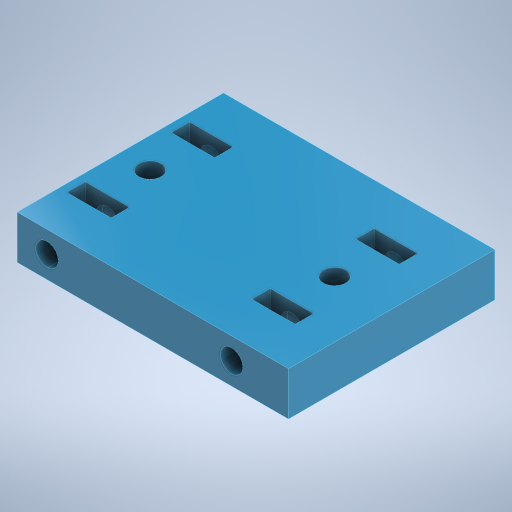
# Autodesk Inventor part: 3D_upper_to_head1
Saved by Autodesk Inventor 2024 (Build 280153000, 153)
## iProperties
Created: 2024-09-08
Part Number: 3D_upper_to_head1
Material: 일반
Document SubType Name: Modeling
Designer: jmha0
Density: 1 g/cm^3
Appearance: 하늘색 짙음
Author: jmha0
Autodesk Inventor part; units mm, degrees
ref_plane "YZ Plane" through (0, 0, 0) normal (1, 0, 0) x (0, 1, 0)
ref_plane "XZ Plane" through (0, 0, 0) normal (0, 1, 0) x (-1, 0, 0)
ref_plane "XY Plane" through (0, 0, 0) normal (0, 0, 1) x (1, 0, 0)
sketch "스케치1" plane through (0, 0, 0) normal (0, 1, 0) x (-1, 0, 0)
  line L0 (206.554, -381.1375) -> (206.9537, -381.1375)
  line L1 (206.9537, -381.1375) -> (207.1542, -381.1375)
  line L2 (207.1542, -381.1375) -> (210.304, -381.1375)
  line L3 (210.304, -381.1375) -> (210.304, -370.6375)
  line L4 (210.304, -370.6375) -> (211.404, -370.6375)
  line L5 (211.404, -370.6375) -> (211.404, -356.1375)
  line L6 (211.404, -356.1375) -> (224.204, -356.1375)
  line L7 (224.204, -370.6375) -> (224.204, -356.1375)
  line L8 (224.204, -370.6375) -> (225.304, -370.6375)
  line L9 (225.304, -381.1375) -> (225.304, -370.6375)
  line L10 (225.304, -381.1375) -> (228.9537, -381.1375)
  line L11 (228.9537, -381.1375) -> (229.1542, -381.1375)
  line L12 (229.1542, -381.1375) -> (233.029, -381.1375)
  line L13 (233.029, -383.6375) -> (233.029, -381.1375)
  line L14 (233.029, -383.6375) -> (247.079, -383.6375)
  line L15 (247.079, -383.6375) -> (247.079, -381.1375)
  line L16 (247.079, -381.1375) -> (250.9537, -381.1375)
  line L17 (250.9537, -381.1375) -> (251.1542, -381.1375)
  line L18 (251.1542, -381.1375) -> (255.029, -381.1375)
  line L19 (255.029, -383.6375) -> (255.029, -381.1375)
  line L20 (255.029, -383.6375) -> (258.054, -383.6375)
  line L21 (258.054, -353.6375) -> (258.054, -383.6375)
  line L22 (255.029, -353.6375) -> (258.054, -353.6375)
  line L23 (255.029, -353.6375) -> (255.029, -356.1375)
  line L24 (251.1542, -356.1375) -> (255.029, -356.1375)
  line L25 (250.9537, -356.1375) -> (251.1542, -356.1375)
  line L26 (247.079, -356.1375) -> (250.9537, -356.1375)
  line L27 (247.079, -353.6375) -> (247.079, -356.1375)
  line L28 (233.029, -353.6375) -> (247.079, -353.6375)
  line L29 (233.029, -353.6375) -> (233.029, -356.1375)
  line L30 (229.1542, -356.1375) -> (233.029, -356.1375)
  line L31 (228.9537, -356.1375) -> (229.1542, -356.1375)
  line L32 (225.079, -356.1375) -> (228.9537, -356.1375)
  line L33 (225.079, -353.6375) -> (225.079, -356.1375)
  line L34 (211.029, -353.6375) -> (225.079, -353.6375)
  line L35 (211.029, -353.6375) -> (211.029, -356.1375)
  line L36 (207.1542, -356.1375) -> (211.029, -356.1375)
  line L37 (206.9537, -356.1375) -> (207.1542, -356.1375)
  line L38 (206.554, -356.1375) -> (206.9537, -356.1375)
  line L39 (206.554, -356.1375) -> (206.554, -381.1375)
  circle A0 centre (240.054, -368.6375) radius 5.2901
  line L40 (258.054, -356.1375) -> (225.304, -356.1375)
  line L41 (225.304, -356.1375) -> (225.304, -381.1375)
  line L42 (225.304, -381.1375) -> (258.054, -381.1375)
  line L43 (258.054, -381.1375) -> (258.054, -356.1375)
  line L44 (257.854, -356.3375) -> (225.504, -356.3375)
  line L45 (225.504, -356.3375) -> (225.504, -380.9375)
  line L46 (225.504, -380.9375) -> (257.854, -380.9375)
  line L47 (257.854, -380.9375) -> (257.854, -356.3375)
  line L48 (255.029, -354.8875) -> (251.054, -354.8875)
  circle A1 centre (251.054, -354.8875) radius 0.8707
  line L49 (255.029, -382.3875) -> (247.079, -382.3875)
  line L50 (251.054, -354.8875) -> (251.054, -382.3875)
  line L51 (233.029, -354.8875) -> (229.054, -354.8875)
  line L52 (229.054, -354.8875) -> (229.054, -382.3875)
  dimension "d37" = 25
  dimension "d38" = 32.75
  dimension "d39" = 0.2
  dimension "d40" = 2.5
  dimension "d41" = 7.95
  dimension "d42" = 3.975
  dimension "d43" = 3.975
  constraints: 106 end point, 5 midpoint, 5 parallel, 3 perpendicular, 2 centre point, 2 horizontal, 1 coincident, 1 point on line, 3 other
  measures "d37" distance of L18.end L24.end
  measures "d38" distance from line of L21 L9.start
  measures "d39" distance between parallel lines of L43 L47
  measures "d40" distance of L22.start L24.end
  measures "d41" distance between parallel lines of L27 L23
  measures "d42" distance of L48.start L48.end
  measures "d43" distance of L51.start L51.end
extrude "돌출2" add sketch "스케치1" along normal blind 5.2 contours L52 L46 L45 L44 | L44 L50 L46 L52 | L44 L47 L46 L50 | A0
sketch "스케치4" plane through (-225.504, 0, -380.9375) normal (0, 0, -1) x (-1, 0, 0)
  line L0 (0, 0) -> (32.35, 0) projected
  line L1 (32.35, 0) -> (32.35, 5.2) projected
  line L2 (0, 5.2) -> (32.35, 5.2) projected
  line L3 (0, 0) -> (0, 5.2) projected
  line L4 (32.35, 5.2) -> (28.8, 5.2)
  line L5 (32.35, 5.2) -> (0, 5.2) projected
  line L6 (0, 5.2) -> (6.8, 5.2)
  line L7 (32.35, 2.6) -> (0, 2.6)
  circle A0 centre (28.8, 2.6) radius 1.35
  circle A1 centre (6.8, 2.6) radius 1.35
  point P0 (-225.504, 0)
  dimension "d59" = 3.55
  dimension "d60" = 6.8
  dimension "d69" = 2.7
  dimension "d70" = 2.7
  constraints: 6 end point, 4 point on line, 2 centre point, 2 midpoint
  measures "d59" distance of L1.end L4.end
  measures "d60" distance of L2.start L6.end
  measures "d69" diameter of A0
  measures "d70" diameter of A1
extrude "돌출3" cut sketch "스케치4" against normal blind 8 contours A1 L7 | L7 A1 | A0 L7 | L7 A0
sketch "스케치5" plane through (-257.854, 0, -356.3375) normal (0, 0, 1) x (1, 0, 0)
  circle A0 centre (3.55, 3) radius 1.35 projected
  circle A1 centre (25.55, 3) radius 1.35 projected
  circle A2 centre (3.55, 2.6) radius 1.35 projected
  circle A3 centre (25.55, 2.6) radius 1.35 projected
  point P0 (257.854, 0)
extrude "돌출4" cut sketch "스케치5" against normal blind 8 contours A2 A0 | A0 A2 | A3 A1 | A1 A3 picked at (3.4443, 2.4292) picked at (3.7277, 1.535) picked at (25.4443, 2.4292) picked at (25.7277, 1.535)
sketch "스케치6" plane through (0, 0, 0) normal (0, -1, 0) x (1, 0, 0)
  line L0 (-225.504, -356.3375) -> (-225.504, -380.9375) projected
  line L1 (-225.504, -356.3375) -> (-225.504, -380.9375) projected
  line L2 (-225.504, -356.3375) -> (-225.504, -380.9375) projected
  line L3 (-225.504, -356.3375) -> (-225.504, -380.9375) projected
  line L4 (-257.854, -356.3375) -> (-225.504, -356.3375) projected
  line L5 (-230.954, -380.9375) -> (-233.654, -380.9375) projected
  line L6 (-230.954, -372.9375) -> (-233.654, -372.9375) projected
  line L7 (-233.654, -356.3375) -> (-230.954, -356.3375) projected
  line L8 (-233.654, -364.3375) -> (-230.954, -364.3375) projected
  line L9 (-230.954, -372.9375) -> (-233.654, -372.9375) projected
  line L10 (-230.954, -372.9375) -> (-233.654, -372.9375) projected
  line L11 (-230.954, -380.9375) -> (-233.654, -380.9375) projected
  line L12 (-233.654, -364.3375) -> (-230.954, -364.3375) projected
  line L13 (-233.654, -364.3375) -> (-230.954, -364.3375) projected
  line L14 (-233.654, -356.3375) -> (-230.954, -356.3375) projected
  line L15 (-255.654, -356.3375) -> (-252.954, -356.3375) projected
  line L16 (-255.654, -364.3375) -> (-252.954, -364.3375) projected
  line L17 (-255.654, -356.3375) -> (-252.954, -356.3375) projected
  line L18 (-257.854, -356.3375) -> (-225.504, -356.3375) projected
  line L19 (-257.854, -380.9375) -> (-257.854, -356.3375) projected
  line L20 (-257.854, -380.9375) -> (-257.854, -356.3375) projected
  line L21 (-257.854, -356.3375) -> (-225.504, -356.3375) projected
  line L22 (-257.854, -380.9375) -> (-257.854, -356.3375) projected
  line L23 (-225.504, -380.9375) -> (-257.854, -380.9375) projected
  line L24 (-225.504, -356.3375) -> (-225.504, -380.9375) projected
  line L25 (-257.854, -356.3375) -> (-225.504, -356.3375) projected
  line L26 (-225.504, -356.3375) -> (-225.504, -380.9375) projected
  line L27 (-225.504, -380.9375) -> (-257.854, -380.9375) projected
  line L28 (-257.854, -380.9375) -> (-257.854, -356.3375) projected
  line L29 (-257.854, -356.3375) -> (-225.504, -356.3375) projected
  line L30 (-257.854, -356.3375) -> (-225.504, -356.3375) projected
  line L31 (-257.854, -380.9375) -> (-257.854, -356.3375) projected
  line L32 (-257.854, -380.9375) -> (-257.854, -356.3375) projected
  line L33 (-255.654, -364.3375) -> (-252.954, -364.3375) projected
  line L34 (-255.654, -364.3375) -> (-252.954, -364.3375) projected
  line L35 (-252.954, -372.9375) -> (-255.654, -372.9375) projected
  line L36 (-252.954, -372.9375) -> (-255.654, -372.9375) projected
  line L37 (-252.954, -372.9375) -> (-255.654, -372.9375) projected
  line L38 (-252.954, -380.9375) -> (-255.654, -380.9375) projected
  line L39 (-252.954, -380.9375) -> (-255.654, -380.9375) projected
  line L40 (-225.504, -380.9375) -> (-257.854, -380.9375) projected
  line L41 (-225.504, -380.9375) -> (-257.854, -380.9375) projected
  line L42 (-225.504, -380.9375) -> (-257.854, -380.9375) projected
  line L43 (-225.504, -380.9375) -> (-257.854, -380.9375) projected
  line L44 (-252.954, -356.3375) -> (-252.954, -364.3375) projected
  line L45 (-255.654, -356.3375) -> (-255.654, -364.3375) projected
  line L46 (-255.654, -380.9375) -> (-255.654, -372.9375) projected
  line L47 (-252.954, -380.9375) -> (-252.954, -372.9375) projected
  line L48 (-233.654, -380.9375) -> (-233.654, -372.9375) projected
  line L49 (-230.954, -380.9375) -> (-230.954, -372.9375) projected
  line L50 (-233.654, -356.3375) -> (-233.654, -364.3375) projected
  line L51 (-230.954, -356.3375) -> (-230.954, -364.3375) projected
  line L52 (-232.304, -365.7508) -> (-231.054, -366.4725)
  line L53 (-233.554, -366.4725) -> (-232.304, -365.7508)
  line L54 (-229.804, -367.1941) -> (-229.804, -368.6375)
  line L55 (-231.054, -366.4725) -> (-229.804, -367.1941)
  line L56 (-234.804, -368.6375) -> (-234.804, -367.1941)
  line L57 (-234.804, -367.1941) -> (-233.554, -366.4725)
  line L58 (-234.804, -368.6375) -> (-234.804, -367.1941)
  line L59 (-234.804, -370.0809) -> (-234.804, -368.6375)
  line L60 (-231.054, -370.8026) -> (-232.304, -371.5243)
  line L61 (-232.304, -371.5243) -> (-233.554, -370.8026)
  line L62 (-229.804, -368.6375) -> (-229.804, -370.0809)
  line L63 (-229.804, -370.0809) -> (-231.054, -370.8026)
  line L64 (-229.804, -367.1941) -> (-229.804, -368.6375)
  line L65 (-231.054, -366.4725) -> (-229.804, -367.1941)
  line L66 (-233.554, -370.8026) -> (-234.804, -370.0809)
  line L67 (-234.804, -370.0809) -> (-234.804, -368.6375)
  line L68 (-254.304, -365.7508) -> (-253.054, -366.4725)
  line L69 (-255.554, -366.4725) -> (-254.304, -365.7508)
  line L70 (-251.804, -367.1941) -> (-251.804, -368.6375)
  line L71 (-253.054, -366.4725) -> (-251.804, -367.1941)
  line L72 (-256.804, -368.6375) -> (-256.804, -367.1941)
  line L73 (-256.804, -367.1941) -> (-255.554, -366.4725)
  line L74 (-256.804, -368.6375) -> (-256.804, -367.1941)
  line L75 (-256.804, -370.0809) -> (-256.804, -368.6375)
  line L76 (-253.054, -370.8026) -> (-254.304, -371.5243)
  line L77 (-254.304, -371.5243) -> (-255.554, -370.8026)
  line L78 (-251.804, -368.6375) -> (-251.804, -370.0809)
  line L79 (-251.804, -370.0809) -> (-253.054, -370.8026)
  line L80 (-251.804, -367.1941) -> (-251.804, -368.6375)
  line L81 (-253.054, -366.4725) -> (-251.804, -367.1941)
  line L82 (-255.554, -370.8026) -> (-256.804, -370.0809)
  line L83 (-256.804, -370.0809) -> (-256.804, -368.6375)
  point P0 (0, 0)
  point P1 (-232.304, -368.6375)
  point P2 (-254.304, -368.6375)
  dimension "d75" = 5.7735
  constraints: 64 end point, 4 other
  measures "d75" distance of L68.start L77.start
extrude "돌출5" cut sketch "스케치6" against normal blind 2 contours L52 L55 L54 L62 L63 L60 L61 L66 L59 L56 L57 L53 | L68 L71 L70 L78 L79 L76 L77 L82 L75 L72 L73 L69
sketch "스케치7" plane through (0, 2, 0) normal (0, -1, 0) x (1, 0, 0)
  line L0 (-256.804, -367.1941) -> (-254.304, -365.7508) projected
  line L1 (-256.804, -370.0809) -> (-256.804, -367.1941) projected
  line L2 (-254.304, -371.5243) -> (-256.804, -370.0809) projected
  line L3 (-251.804, -370.0809) -> (-254.304, -371.5243) projected
  line L4 (-251.804, -367.1941) -> (-251.804, -370.0809) projected
  line L5 (-254.304, -365.7508) -> (-251.804, -367.1941) projected
  line L6 (-234.804, -367.1941) -> (-232.304, -365.7508) projected
  line L7 (-234.804, -370.0809) -> (-234.804, -367.1941) projected
  line L8 (-232.304, -371.5243) -> (-234.804, -370.0809) projected
  line L9 (-229.804, -370.0809) -> (-232.304, -371.5243) projected
  line L10 (-229.804, -367.1941) -> (-229.804, -370.0809) projected
  line L11 (-232.304, -365.7508) -> (-229.804, -367.1941) projected
  circle A0 centre (-254.2813, -368.5983) radius 1.35
  circle A1 centre (-232.2869, -368.608) radius 1.35
  point P0 (0, 0)
  dimension "d71" = 2.7
  dimension "d72" = 2.7
  constraints: 2 centre point
  measures "d71" diameter of A0
  measures "d72" diameter of A1
extrude "돌출6" cut sketch "스케치7" against normal blind 8 contours A0 | A1
sketch "스케치9" plane through (0, 0, 0) normal (0, -1, 0) x (1, 0, 0)
  circle A0 centre (-232.2869, -368.608) radius 1.35 projected
  line L0 (-234.804, -367.1941) -> (-232.304, -365.7508) projected
  line L1 (-234.804, -370.0809) -> (-234.804, -367.1941) projected
  line L2 (-232.304, -371.5243) -> (-234.804, -370.0809) projected
  line L3 (-229.804, -370.0809) -> (-232.304, -371.5243) projected
  line L4 (-229.804, -367.1941) -> (-229.804, -370.0809) projected
  line L5 (-232.304, -365.7508) -> (-229.804, -367.1941) projected
  circle A1 centre (-254.2813, -368.5983) radius 1.35 projected
  line L6 (-256.804, -367.1941) -> (-254.304, -365.7508) projected
  line L7 (-256.804, -370.0809) -> (-256.804, -367.1941) projected
  line L8 (-254.304, -371.5243) -> (-256.804, -370.0809) projected
  line L9 (-251.804, -370.0809) -> (-254.304, -371.5243) projected
  line L10 (-251.804, -367.1941) -> (-251.804, -370.0809) projected
  line L11 (-254.304, -365.7508) -> (-251.804, -367.1941) projected
  line L12 (-251.704, -367.1364) -> (-251.704, -370.1386)
  line L13 (-251.704, -370.1386) -> (-254.304, -371.6397)
  line L14 (-254.304, -371.6397) -> (-256.904, -370.1386)
  line L15 (-256.904, -370.1386) -> (-256.904, -367.1364)
  line L16 (-256.904, -367.1364) -> (-254.304, -365.6353)
  line L17 (-254.304, -365.6353) -> (-251.704, -367.1364)
  line L18 (-232.304, -365.6353) -> (-234.904, -367.1364)
  line L19 (-234.904, -367.1364) -> (-234.904, -370.1386)
  line L20 (-234.904, -370.1386) -> (-232.304, -371.6397)
  line L21 (-232.304, -371.6397) -> (-229.704, -370.1386)
  line L22 (-229.704, -370.1386) -> (-229.704, -367.1364)
  line L23 (-229.704, -367.1364) -> (-232.304, -365.6353)
  point P0 (0, 0)
  dimension "d78" = 0.1
  dimension "d79" = 0.1
  constraints: 24 end point, 10 other
  measures "d78" distance between parallel lines of L11 L17
  measures "d79" distance between parallel lines of L0 L18
extrude "돌출7" cut sketch "스케치9" against normal blind 2.2 contours A0 | L0 L5 L4 L3 L2 L1 | A1 | L6 L11 L10 L9 L8 L7 | L12 L13 L14 L15 L16 L17 | L23 L22 L21 L20 L19 L18
sketch "스케치10" plane through (0, 0, 0) normal (0, -1, 0) x (1, 0, 0)
  line L0 (-252.954, -380.9375) -> (-255.654, -380.9375) projected
  line L1 (-257.854, -380.9375) -> (-257.854, -356.3375) projected
  line L2 (-257.854, -380.9375) -> (-257.854, -356.3375) projected
  line L3 (-255.654, -356.3375) -> (-252.954, -356.3375) projected
  line L4 (-252.954, -372.9375) -> (-255.654, -372.9375) projected
  line L5 (-255.654, -364.3375) -> (-252.954, -364.3375) projected
  circle A0 centre (-254.2813, -368.5983) radius 1.35 projected
  line L6 (-230.954, -380.9375) -> (-233.654, -380.9375) projected
  line L7 (-230.954, -372.9375) -> (-233.654, -372.9375) projected
  line L8 (-230.954, -372.9375) -> (-233.654, -372.9375) projected
  line L9 (-230.954, -372.9375) -> (-233.654, -372.9375) projected
  line L10 (-230.954, -380.9375) -> (-233.654, -380.9375) projected
  line L11 (-233.654, -364.3375) -> (-230.954, -364.3375) projected
  line L12 (-233.654, -364.3375) -> (-230.954, -364.3375) projected
  line L13 (-233.654, -356.3375) -> (-230.954, -356.3375) projected
  line L14 (-233.654, -364.3375) -> (-230.954, -364.3375) projected
  line L15 (-233.654, -356.3375) -> (-230.954, -356.3375) projected
  line L16 (-257.854, -356.3375) -> (-225.504, -356.3375) projected
  line L17 (-257.854, -356.3375) -> (-225.504, -356.3375) projected
  line L18 (-225.504, -356.3375) -> (-225.504, -380.9375) projected
  line L19 (-225.504, -356.3375) -> (-225.504, -380.9375) projected
  line L20 (-225.504, -380.9375) -> (-257.854, -380.9375) projected
  line L21 (-225.504, -380.9375) -> (-257.854, -380.9375) projected
  line L22 (-230.954, -380.9375) -> (-233.654, -380.9375) projected
  line L23 (-252.954, -380.9375) -> (-255.654, -380.9375) projected
  line L24 (-225.504, -380.9375) -> (-257.854, -380.9375) projected
  line L25 (-225.504, -380.9375) -> (-257.854, -380.9375) projected
  line L26 (-256.904, -370.1386) -> (-256.904, -367.1364) projected
  line L27 (-256.904, -367.1364) -> (-254.304, -365.6353) projected
  line L28 (-254.304, -365.6353) -> (-251.704, -367.1364) projected
  line L29 (-251.704, -367.1364) -> (-251.704, -370.1386) projected
  line L30 (-251.704, -370.1386) -> (-254.304, -371.6397) projected
  line L31 (-254.304, -371.6397) -> (-256.904, -370.1386) projected
  line L32 (-232.304, -371.6397) -> (-234.904, -370.1386) projected
  line L33 (-234.904, -370.1386) -> (-234.904, -367.1364) projected
  line L34 (-234.904, -367.1364) -> (-232.304, -365.6353) projected
  line L35 (-232.304, -365.6353) -> (-229.704, -367.1364) projected
  line L36 (-229.704, -367.1364) -> (-229.704, -370.1386) projected
  line L37 (-229.704, -370.1386) -> (-232.304, -371.6397) projected
  line L38 (-257.854, -356.3375) -> (-225.504, -356.3375) projected
  line L39 (-257.854, -380.9375) -> (-257.854, -356.3375) projected
  line L40 (-225.504, -380.9375) -> (-257.854, -380.9375) projected
  line L41 (-225.504, -356.3375) -> (-225.504, -380.9375) projected
  circle A1 centre (-232.2869, -368.608) radius 1.35 projected
  circle A2 centre (-254.2813, -368.5983) radius 1.35 projected
  line L42 (-257.854, -356.3375) -> (-225.504, -356.3375) projected
  line L43 (-225.504, -356.3375) -> (-225.504, -380.9375) projected
  line L44 (-225.504, -380.9375) -> (-257.854, -380.9375) projected
  line L45 (-257.854, -380.9375) -> (-257.854, -356.3375) projected
  line L46 (-233.654, -356.3375) -> (-230.954, -356.3375) projected
  line L47 (-255.654, -356.3375) -> (-252.954, -356.3375) projected
  line L48 (-257.854, -356.3375) -> (-225.504, -356.3375) projected
  line L49 (-257.854, -356.3375) -> (-225.504, -356.3375) projected
  line L50 (-234.904, -370.1386) -> (-234.904, -367.1364) projected
  line L51 (-234.904, -370.1386) -> (-234.904, -367.1364) projected
  line L52 (-232.304, -371.6397) -> (-234.904, -370.1386) projected
  line L53 (-232.304, -371.6397) -> (-234.904, -370.1386) projected
  line L54 (-232.304, -371.6397) -> (-234.904, -370.1386) projected
  line L55 (-232.304, -371.6397) -> (-234.904, -370.1386) projected
  line L56 (-234.904, -367.1364) -> (-232.304, -365.6353) projected
  line L57 (-234.904, -367.1364) -> (-232.304, -365.6353) projected
  line L58 (-234.904, -367.1364) -> (-232.304, -365.6353) projected
  line L59 (-234.904, -367.1364) -> (-232.304, -365.6353) projected
  circle A3 centre (-232.2869, -368.608) radius 1.35 projected
  circle A4 centre (-232.2869, -368.608) radius 1.35 projected
  circle A5 centre (-232.2869, -368.608) radius 1.35 projected
  circle A6 centre (-232.2869, -368.608) radius 1.35 projected
  line L60 (-234.904, -370.1386) -> (-234.904, -367.1364) projected
  line L61 (-232.304, -371.6397) -> (-234.904, -370.1386) projected
  line L62 (-229.704, -370.1386) -> (-232.304, -371.6397) projected
  line L63 (-229.704, -367.1364) -> (-229.704, -370.1386) projected
  line L64 (-232.304, -365.6353) -> (-229.704, -367.1364) projected
  line L65 (-234.904, -367.1364) -> (-232.304, -365.6353) projected
  line L66 (-229.704, -367.1364) -> (-229.704, -370.1386) projected
  line L67 (-229.704, -367.1364) -> (-229.704, -370.1386) projected
  line L68 (-229.704, -367.1364) -> (-229.704, -370.1386) projected
  line L69 (-232.304, -365.6353) -> (-229.704, -367.1364) projected
  line L70 (-232.304, -365.6353) -> (-229.704, -367.1364) projected
  line L71 (-225.504, -356.3375) -> (-225.504, -380.9375) projected
  line L72 (-225.504, -356.3375) -> (-225.504, -380.9375) projected
  circle A7 centre (-232.2869, -368.608) radius 1.35 projected
  line L73 (-232.304, -365.6353) -> (-229.704, -367.1364) projected
  line L74 (-229.704, -367.1364) -> (-229.704, -370.1386) projected
  line L75 (-229.704, -370.1386) -> (-232.304, -371.6397) projected
  line L76 (-232.304, -365.6353) -> (-229.704, -367.1364) projected
  line L77 (-229.704, -370.1386) -> (-232.304, -371.6397) projected
  line L78 (-229.704, -370.1386) -> (-232.304, -371.6397) projected
  line L79 (-229.704, -370.1386) -> (-232.304, -371.6397) projected
  line L80 (-234.904, -370.1386) -> (-234.904, -367.1364) projected
  line L81 (-251.704, -367.1364) -> (-251.704, -370.1386) projected
  line L82 (-251.704, -367.1364) -> (-251.704, -370.1386) projected
  line L83 (-254.304, -365.6353) -> (-251.704, -367.1364) projected
  line L84 (-254.304, -365.6353) -> (-251.704, -367.1364) projected
  line L85 (-251.704, -370.1386) -> (-254.304, -371.6397) projected
  line L86 (-251.704, -370.1386) -> (-254.304, -371.6397) projected
  circle A8 centre (-254.2813, -368.5983) radius 1.35 projected
  line L87 (-256.904, -367.1364) -> (-254.304, -365.6353) projected
  line L88 (-256.904, -367.1364) -> (-254.304, -365.6353) projected
  line L89 (-254.304, -371.6397) -> (-256.904, -370.1386) projected
  line L90 (-254.304, -371.6397) -> (-256.904, -370.1386) projected
  line L91 (-234.904, -370.1386) -> (-234.904, -367.1364) projected
  line L92 (-251.704, -370.1386) -> (-254.304, -371.6397) projected
  line L93 (-251.704, -370.1386) -> (-254.304, -371.6397) projected
  line L94 (-252.954, -372.9375) -> (-255.654, -372.9375) projected
  line L95 (-252.954, -372.9375) -> (-255.654, -372.9375) projected
  line L96 (-252.954, -380.9375) -> (-255.654, -380.9375) projected
  line L97 (-254.304, -365.6353) -> (-251.704, -367.1364) projected
  line L98 (-254.304, -365.6353) -> (-251.704, -367.1364) projected
  line L99 (-254.304, -371.6397) -> (-256.904, -370.1386) projected
  line L100 (-254.304, -371.6397) -> (-256.904, -370.1386) projected
  circle A9 centre (-254.2813, -368.5983) radius 1.35 projected
  circle A10 centre (-254.2813, -368.5983) radius 1.35 projected
  line L101 (-256.904, -370.1386) -> (-256.904, -367.1364) projected
  line L102 (-256.904, -370.1386) -> (-256.904, -367.1364) projected
  line L103 (-256.904, -370.1386) -> (-256.904, -367.1364) projected
  line L104 (-256.904, -370.1386) -> (-256.904, -367.1364) projected
  line L105 (-255.654, -364.3375) -> (-252.954, -364.3375) projected
  circle A11 centre (-254.2813, -368.5983) radius 1.35 projected
  line L106 (-256.904, -367.1364) -> (-254.304, -365.6353) projected
  line L107 (-256.904, -370.1386) -> (-256.904, -367.1364) projected
  line L108 (-254.304, -371.6397) -> (-256.904, -370.1386) projected
  line L109 (-251.704, -370.1386) -> (-254.304, -371.6397) projected
  line L110 (-251.704, -367.1364) -> (-251.704, -370.1386) projected
  line L111 (-254.304, -365.6353) -> (-251.704, -367.1364) projected
  line L112 (-257.854, -380.9375) -> (-257.854, -356.3375) projected
  line L113 (-257.854, -380.9375) -> (-257.854, -356.3375) projected
  line L114 (-256.904, -367.1364) -> (-254.304, -365.6353) projected
  line L115 (-256.904, -367.1364) -> (-254.304, -365.6353) projected
  line L116 (-255.654, -364.3375) -> (-252.954, -364.3375) projected
  line L117 (-255.654, -356.3375) -> (-252.954, -356.3375) projected
  line L118 (-251.704, -367.1364) -> (-251.704, -370.1386) projected
  line L119 (-251.704, -367.1364) -> (-251.704, -370.1386) projected
  line L120 (-252.954, -380.9375) -> (-252.954, -372.9375) projected
  line L121 (-255.654, -380.9375) -> (-255.654, -372.9375) projected
  line L122 (-255.654, -356.3375) -> (-255.654, -364.3375) projected
  line L123 (-252.954, -356.3375) -> (-252.954, -364.3375) projected
  line L124 (-233.654, -380.9375) -> (-233.654, -372.9375) projected
  line L125 (-230.954, -380.9375) -> (-230.954, -372.9375) projected
  line L126 (-233.654, -356.3375) -> (-233.654, -364.3375) projected
  line L127 (-230.954, -356.3375) -> (-230.954, -364.3375) projected
  line L128 (-254.304, -380.9375) -> (-254.304, -374.8375)
  line L129 (-251.704, -375.9375) -> (-256.904, -375.9375)
  line L130 (-256.904, -375.9375) -> (-256.904, -373.7375)
  line L131 (-256.904, -373.7375) -> (-251.704, -373.7375)
  line L132 (-251.704, -373.7375) -> (-251.704, -375.9375)
  line L133 (-251.704, -375.9375) -> (-256.904, -373.7375) construction
  line L134 (-256.904, -375.9375) -> (-251.704, -373.7375) construction
  line L135 (-234.904, -375.9375) -> (-229.704, -375.9375)
  line L136 (-229.704, -375.9375) -> (-229.704, -373.7375)
  line L137 (-229.704, -373.7375) -> (-234.904, -373.7375)
  line L138 (-234.904, -373.7375) -> (-234.904, -375.9375)
  line L139 (-234.904, -375.9375) -> (-229.704, -373.7375) construction
  line L140 (-229.704, -375.9375) -> (-234.904, -373.7375) construction
  line L141 (-254.304, -356.3375) -> (-254.304, -362.4375)
  line L142 (-251.6578, -363.5375) -> (-256.9501, -363.5375)
  line L143 (-256.9501, -363.5375) -> (-256.9501, -361.3375)
  line L144 (-256.9501, -361.3375) -> (-251.6578, -361.3375)
  line L145 (-251.6578, -361.3375) -> (-251.6578, -363.5375)
  line L146 (-251.6578, -363.5375) -> (-256.9501, -361.3375) construction
  line L147 (-256.9501, -363.5375) -> (-251.6578, -361.3375) construction
  line L148 (-229.704, -363.5375) -> (-234.904, -363.5375)
  line L149 (-234.904, -363.5375) -> (-234.904, -361.3375)
  line L150 (-234.904, -361.3375) -> (-229.704, -361.3375)
  line L151 (-229.704, -361.3375) -> (-229.704, -363.5375)
  line L152 (-229.704, -363.5375) -> (-234.904, -361.3375) construction
  line L153 (-234.904, -363.5375) -> (-229.704, -361.3375) construction
  point P0 (0, 0)
  point P1 (-232.304, -374.8375)
  point P2 (-232.304, -362.4375)
  dimension "d82" = 6.1
  dimension "d83" = 5.2
  dimension "d84" = 2.2
  dimension "d85" = 5.2
  dimension "d86" = 2.2
  dimension "d87" = 6.1
  dimension "d88" = 2.2
  dimension "d89" = 2.2
  constraints: 52 end point, 10 midpoint, 9 parallel, 4 horizontal, 4 perpendicular, 1 vertical, 5 other
  measures "d82" distance of L128.start L128.end
  measures "d83" distance of L130.end L131.end
  measures "d84" distance of L129.end L130.end
  measures "d85" distance of L137.end L136.end
  measures "d86" distance of L136.end L135.end
  measures "d87" distance of L141.start L141.end
  measures "d88" distance of L142.end L143.end
  measures "d89" distance of L148.end L149.end
extrude "돌출8" cut sketch "스케치10" against normal blind 6 contours L129 L121 L131 L120 | L120 L131 L132 L129 | L135 L138 L137 L124 | L124 L137 L125 L135 | L129 L130 L131 L121 | L125 L137 L136 L135 | L144 L123 L142 L122 | L122 L142 L143 L144 | L150 L151 L148 L127 | L127 L148 L126 L150 | L126 L148 L149 L150 | L144 L145 L142 L123
